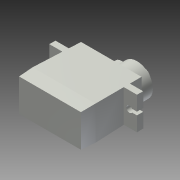
# Autodesk Inventor part: servo
Saved by Autodesk Inventor 2015 (Build 190159000, 159)
## iProperties
Created: 2014-07-17
Part Number: servo
Material: ABS Plastic
Document SubType Name: Modeling
Designer: Sebastian
Density: 1.06 g/cm^3
Appearance: Smooth - White
Author: Sebastian
Autodesk Inventor part; units mm, degrees
sketch "Sketch1" plane through (0, 0, 0) normal (0, 1, 0) x (-1, 0, 0)
  line L0 (0, 0) -> (22.8, 0)
  line L1 (22.8, 0) -> (22.8, -12)
  line L2 (22.8, -12) -> (0, -12)
  line L3 (0, -12) -> (0, 0)
  dimension "d0" = 22.8
  dimension "d1" = 12
  constraints: 8 end point, 2 parallel, 1 horizontal, 1 perpendicular
  measures "d0" distance of L1.end L2.end
  measures "d1" distance of L0.end L1.end
ref_plane "Work Plane3" through (0, 5.2, 0) normal (0, 1, 0) x (-1, 0, 0)
sketch "Sketch5" plane through (0, 5.2, 0) normal (0, 1, 0) x (-1, 0, 0)
  line L0 (11.4, -12.25) -> (23, -12.25)
  line L1 (23, -12.25) -> (-0.2, -12.25)
  line L2 (-0.2, -12.25) -> (-0.2, 0.25)
  line L3 (-0.2, 0.25) -> (23, 0.25)
  line L4 (23, 0.25) -> (23, -12.25)
  dimension "d32" = 23.2
  dimension "d33" = 12.5
  constraints: 10 end point, 2 horizontal, 2 parallel, 1 perpendicular
  measures "d32" distance of L2.end L3.end
  measures "d33" distance of L1.end L2.end
sketch "Sketch1 outline for Loft1" plane through (0, 0, 0) normal (0, 1, 0) x (-1, 0, 0)
  line L0 (0, 0) -> (22.8, 0)
  line L1 (22.8, 0) -> (22.8, -12)
  line L2 (22.8, -12) -> (0, -12)
  line L3 (0, -12) -> (0, 0)
sketch "Sketch5 outline for Loft1" plane through (0, 5.2, 0) normal (0, 1, 0) x (-1, 0, 0)
  line L0 (23, -12.25) -> (-0.2, -12.25)
  line L1 (-0.2, -12.25) -> (-0.2, 0.25)
  line L2 (-0.2, 0.25) -> (23, 0.25)
  line L3 (23, 0.25) -> (23, -12.25)
loft "Loft1" add profiles "Sketch1 outline for Loft1", "Sketch5 outline for Loft1"
ref_plane "Work Plane4" through (0, 22.6, 0) normal (0, 1, 0) x (-1, 0, 0)
sketch "Sketch7" plane through (0, 22.6, 0) normal (0, 1, 0) x (-1, 0, 0)
  line L0 (0.25, -6) -> (0.25, -0.15)
  line L1 (0.25, -0.15) -> (0.25, -11.85)
  line L2 (0.25, -11.85) -> (22.55, -11.85)
  line L3 (0.25, -11.85) -> (22.55, -11.85)
  line L4 (22.55, -11.85) -> (22.55, -0.15)
  line L5 (22.55, -0.15) -> (0.25, -0.15)
  line L6 (0.25, -0.15) -> (0.25, -11.85)
  point P0 (0, 0)
  constraints: 14 end point, 2 parallel, 1 horizontal, 1 perpendicular, 1 vertical
sketch "Sketch7 outline for Loft2" plane through (0, 22.6, 0) normal (0, 1, 0) x (-1, 0, 0)
  line L0 (0.25, -0.15) -> (0.25, -11.85)
  line L1 (22.55, -0.15) -> (0.25, -0.15)
  line L2 (22.55, -11.85) -> (22.55, -0.15)
  line L3 (0.25, -11.85) -> (22.55, -11.85)
loft "Loft2" add profiles "Sketch7 outline for Loft2" section 2 edges at (-11.4, 5.2, 0.25) (0.2, 5.2, -6) (-11.4, 5.2, -12.25) (-23, 5.2, -6)
ref_plane "Work Plane5" through (-11.4, 0, 0) normal (1, 0, 0) x (0, 1, 0)
ref_plane "Work Plane7" through (-0.136245, 18.201471, -0.048884) normal (1, 0, 0) x (0, 1, 0)
ref_plane "Work Plane8" through (-0.136245, 18.201471, -0.048884) normal (-0.0258534, 0.9996657, 0) x (0.9996657, 0.0258534, 0)
sketch "Sketch10" plane through (-0.136245, 18.201471, -0.048884) normal (1, 0, 0) x (0, 1, 0)
  line L0 (0, 0) -> (0, -11.902231)
  line L1 (-2.299231, -11.955087) -> (-2.299231, 0.052856)
  line L2 (4.398529, -0.101116) -> (-13.001471, 0.298884)
  line L3 (4.398529, -11.801116) -> (-13.001471, -12.201116)
  point P0 (-18.201471, 0.048884)
sketch "Sketch10 outline for Extrusion6" plane through (-0.136245, 18.201471, -0.048884) normal (1, 0, 0) x (0, 1, 0)
  line L0 (0, 0) -> (0, -11.902231)
  line L1 (0, -11.902231) -> (-2.299231, -11.955087)
  line L2 (-2.299231, -11.955087) -> (-2.299231, 0.052856)
  line L3 (-2.299231, 0.052856) -> (0, 0)
extrude "Extrusion6" add sketch "Sketch10 outline for Extrusion6" along normal blind 4.9
sketch "Sketch9" plane through (-0.136245, 18.201471, -0.048884) normal (0, 1, 0) x (1, 0, 0)
  arc A0 (3.133494, 6.551116) -> (3.133494, 5.351116) centre (2.151116, 5.951116) ccw
  line L0 (0, 11.902231) -> (4.5, 11.902231)
  line L1 (0, 0) -> (4.5, 0)
  line L2 (0, 0) -> (0, 11.902231)
  line L3 (4.5, 11.902231) -> (4.5, 0)
  line L4 (4.5, 5.951116) -> (4.5, 6.551116)
  line L5 (4.5, 6.551116) -> (3.133494, 6.551116)
  line L6 (3.133494, 6.551116) -> (5.264837, 6.551116)
  line L7 (5.264837, 6.551116) -> (5.264837, 5.351116)
  line L8 (5.264837, 5.351116) -> (3.133494, 5.351116)
  point P0 (-0.334371, -0.048884)
  dimension "d58" = 4.8
  dimension "d59" = 4.8
  dimension "d60" = 1
  dimension "d62" = 1.2
  constraints: 18 end point, 2 point on circle, 1 centre point, 1 horizontal, 1 parallel, 1 perpendicular, 1 point on line
  measures "d58" distance edge to line of A0 L0
  measures "d59" distance edge to line of A0 L1
  measures "d60" distance edge to line of A0 L2
  measures "d62" distance of L6.end L7.end
sketch "Sketch9 outline for Extrusion5" plane through (-0.136245, 18.201471, -0.048884) normal (0, 1, 0) x (1, 0, 0)
  line L0 (5.264837, 6.551116) -> (3.133494, 6.551116)
  line L1 (5.264837, 5.351116) -> (5.264837, 6.551116)
  line L2 (3.133494, 5.351116) -> (5.264837, 5.351116)
  arc A0 (3.133494, 6.551116) -> (3.133494, 5.351116) centre (2.151116, 5.951116) ccw
extrude "Extrusion5" cut sketch "Sketch9 outline for Extrusion5" against normal blind 4.5
mirror "Mirror3" about plane through (-11.4, 0, 0) normal (1, 0, 0) of "Extrusion6", "Extrusion5"
sketch "Sketch11" plane through (-22.55, 22.6, -11.85) normal (0, 1, 0) x (1, 0, 0)
  arc A0 (11.458006, -8.9) -> (11.341184, -3) centre (16.45, -5.85) ccw
  line L0 (22.3, 0) -> (0, 0)
  line L1 (0, -11.7) -> (22.3, -11.7)
  line L2 (22.3, -11.7) -> (22.3, 0)
  arc A1 (10.65, -3) -> (10.65, -8.9) centre (10.65, -5.95) ccw
  line L3 (10.65, -3) -> (11.341184, -3)
  line L4 (10.65, -8.9) -> (11.458006, -8.9)
  point P0 (22.55, -11.85)
  dimension "d68" = 0
  dimension "d69" = 0
  dimension "d70" = 0
  dimension "d71" = 3
  dimension "d72" = 2.8
  dimension "d73" = 14.6
  dimension "d74" = 5.9
  constraints: 4 end point, 4 point on circle, 2 centre point, 2 horizontal, 2 tangent
  measures "d68" distance edge to line of A0 L0
  measures "d69" distance edge to line of A0 L1
  measures "d70" distance edge to line of A0 L2
  measures "d71" distance edge to line of A1 L0
  measures "d72" distance edge to line of A1 L1
  measures "d74" diameter of A1
sketch "Sketch11 outline for Extrusion7" plane through (-22.55, 22.6, -11.85) normal (0, 1, 0) x (1, 0, 0)
  arc A0 (11.341184, -3) -> (11.458006, -8.9) centre (16.45, -5.85) cw
  line L0 (11.458006, -8.9) -> (10.65, -8.9)
  arc A1 (10.65, -8.9) -> (10.65, -3) centre (10.65, -5.95) cw
  line L1 (10.65, -3) -> (11.341184, -3)
extrude "Extrusion7" add sketch "Sketch11 outline for Extrusion7" along normal blind 4.2
sketch "Sketch12" plane through (-22.55, 26.8, -11.85) normal (0, 1, 0) x (1, 0, 0)
  arc A0 (11.458006, -8.9) -> (11.341184, -3) centre (16.45, -5.85) ccw
  circle A1 centre (16.45, -5.85) radius 2.3
  circle A2 centre (16.45, -5.85) radius 0.8
  point P0 (22.55, -11.85)
  dimension "d77" = 4.6
  dimension "d78" = 1.5
  constraints: 2 centre point, 1 coincident
  measures "d77" diameter of A1
  measures "d78" radial gap between concentric circles of A1 A2
sketch "Sketch12 outline for Extrusion8" plane through (-22.55, 26.8, -11.85) normal (0, 1, 0) x (1, 0, 0)
  circle A0 centre (16.45, -5.85) radius 2.3
  circle A1 centre (16.45, -5.85) radius 0.8
extrude "Extrusion8" add sketch "Sketch12 outline for Extrusion8" along normal blind 2.7
ref_plane "Work Plane9" through (-22.55, 26.8, -11.85) normal (0, 1, 0) x (1, 0, 0)
split body "Split1" result two bodies by plane through (-22.55, 26.8, -11.85) normal (0, 1, 0) first body at (-4.305837, 28.6, -5.85516)
body "Solid3"
body "Solid4"
